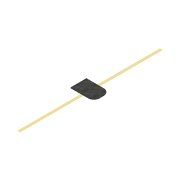
# Autodesk Inventor part: PlacaInferior
Saved by Autodesk Inventor 2021 (Build 250183000, 183)
## iProperties
Created: 2021-05-05
Part Number: PlacaInferior
Material: Steel ASTM A36
Document SubType Name: Modeling
Designer: Santiago Suárez
Mass: 10428.1 g
Surface Area: 2271.44 cm^2
Volume: 1328.41 cm^3
Density: 7.85 g/cm^3
Appearance: Plate
Author: Santiago Suárez
Autodesk Inventor part; units mm, degrees
ref_plane "YZ Plane" through (0, 0, 0) normal (1, 0, 0) x (0, 1, 0)
ref_plane "XZ Plane" through (0, 0, 0) normal (0, 1, 0) x (-1, 0, 0)
ref_plane "XY Plane" through (0, 0, 0) normal (0, 0, 1) x (1, 0, 0)
ref_plane "Work Plane1" through (1104.5696, 91.5553, 211.8164) normal (0, 1, 0) x (-1, 0, 0)
sketch "Sketch1" plane through (1104.5696, 91.5553, 211.8164) normal (0, 1, 0) x (-1, 0, 0)
  arc A0 (57.6551, 1254.9955) -> (57.6551, 1150.0245) centre (104.395, 1202.51) ccw
  line L0 (-26.3951, 1291) -> (133.6049, 1291)
  line L1 (133.6049, 1019) -> (-26.3951, 1019)
  line L2 (-26.3951, 1249) -> (-26.3951, 1291)
  line L3 (179.6049, 2285) -> (179.6049, 25)
  line L4 (179.6049, 1019) -> (179.6049, 1291.0001)
  line L5 (-72.3951, 25) -> (-72.3951, 2285)
  line L6 (179.6049, 1291.0001) -> (-222.3951, 1291.0001)
  line L7 (179.6049, 1019) -> (-222.3951, 1019)
  line L8 (-222.3951, 25) -> (-222.3951, 2285)
  line L9 (-222.3951, 1291.0001) -> (-222.3951, 1019)
  point P0 (1104.5696, -211.8164)
  point P1 (-72.3951, 1291.0001)
  point P2 (-72.3951, 1019)
  point P3 (154, 1291)
  point P4 (4, 1291)
extrude "Extrusion1" add sketch "Sketch1" along normal blind 12.7
sketch "Sketch2" plane through (1104.5696, 104.2553, 211.8164) normal (0, 1, 0) x (1, 0, 0)
  line L0 (222.3951, -1019) -> (-179.6049, -1019) construction
  line L1 (-179.6049, -1019) -> (-179.6049, -1291.0001) construction
  line L2 (-179.6049, -1291.0001) -> (222.3951, -1291.0001) construction
  line L3 (222.3951, -1291.0001) -> (222.3951, -1019) construction
  line L4 (-179.6049, -1291.0001) -> (222.3951, -1291.0001) construction
  line L5 (21.3951, -1291.0001) -> (21.3951, -1019) construction
  line L6 (-179.6049, -1019) -> (-179.6049, -1291.0001) construction
  line L7 (-179.6049, -1155) -> (222.3951, -1155) construction
  point P0 (-1104.5696, 211.8164)
  point P1 (-159.6049, -1266.0001)
  point P2 (50.3951, -1266.0001)
  point P3 (-159.6049, -1044)
  point P4 (50.3951, -1044)
  dimension "d16" = 25
  dimension "d17" = 20
  dimension "d18" = 25
  dimension "d19" = 210
  constraints: 5 midpoint, 4 end point, 2 symmetric about line, 1 perpendicular, 1 point on line
  measures "d16" distance from line of point (-159.605, -1266) L2
  measures "d17" distance from line of point (-159.605, -1266) L1
  measures "d18" distance from line of point (50.395, -1266) L2
  measures "d19" distance of point (-159.605, -1266) point (50.395, -1266)
hole "Hole1" at (944.9647, 104.2553, 1477.8164) at (944.9647, 104.2553, 1255.8164) at (1154.9647, 104.2553, 1255.8164) at (1154.9647, 104.2553, 1477.8164) direction (0, -1, 0) diameter 12 end through all
fillet "Fillet1" radius 100 1 edges at (1326.9647, 97.9053, 1502.8164)
fillet "Fillet2" radius 100 1 edges at (1326.9647, 97.9053, 1230.8164)
body "Solid1"
